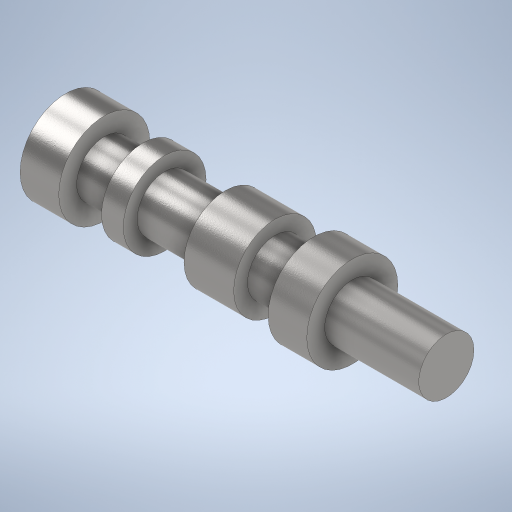
# Autodesk Inventor part: lehrerfreund
Saved by Autodesk Inventor 2024 (Build 280153000, 153)
## iProperties
Created: 2024-02-07
Part Number: lehrerfreund
Material: Stahl, galvanisiert
Document SubType Name: Modeling
Designer: ffogue
Density: 7.85 g/cm^3
Appearance: Galvanisiert
Author: ffogue
Autodesk Inventor part; units mm, degrees
ref_plane "YZ Plane" through (0, 0, 0) normal (1, 0, 0) x (0, 1, 0)
ref_plane "XZ Plane" through (0, 0, 0) normal (0, 1, 0) x (-1, 0, 0)
ref_plane "XY Plane" through (0, 0, 0) normal (0, 0, 1) x (1, 0, 0)
sketch "Skizze1" plane through (0, 0, 0) normal (0, 0, 1) x (1, 0, 0)
  line L0 (0, 0) -> (138, 0)
  line L1 (0, 0) -> (0, 16.5)
  line L2 (0, 16.5) -> (14, 16.5)
  line L3 (14, 16.5) -> (14, 10)
  line L4 (14, 10) -> (28, 10)
  line L5 (28, 10) -> (28, 15)
  line L6 (28, 15) -> (35.9017, 15)
  line L7 (35.9017, 15) -> (35.9017, 10)
  line L8 (35.9017, 10) -> (57.9017, 10)
  line L9 (57.9017, 10) -> (57.9017, 15)
  line L10 (57.9017, 15) -> (75.9017, 15)
  line L11 (75.9017, 15) -> (75.9017, 10)
  line L12 (75.9017, 10) -> (89.9017, 10)
  line L13 (89.9017, 10) -> (89.9017, 16.5)
  line L14 (89.9017, 16.5) -> (103.9017, 16.5)
  line L15 (103.9017, 16.5) -> (103.9017, 10)
  line L16 (103.9017, 10) -> (138, 10)
  line L17 (138, 10) -> (138, 0)
  point P0 (28, 12.5)
  point P1 (103.9017, 13.25)
  point P2 (89.9017, 13.25)
  dimension "d0" = 138
  dimension "d1" = 14
  dimension "d2" = 14
  dimension "d3" = 7.9017
  dimension "d4" = 22
  dimension "d5" = 14
  dimension "d6" = 14
  dimension "d7" = 18
  dimension "d8" = 33
  dimension "d9" = 20
  dimension "d10" = 30
  constraints: 36 end point, 11 perpendicular, 10 point on line, 3 midpoint, 1 coincident, 1 horizontal, 1 vertical
  measures "d0" distance between parallel lines of L17 L1
  measures "d1" distance between parallel lines of L3 L1
  measures "d2" distance from line of point (28, 12.5) L3
  measures "d3" distance between parallel lines of L7 L5
  measures "d4" distance between parallel lines of L9 L7
  measures "d5" distance from line of point (103.902, 13.25) L13
  measures "d6" distance from line of point (89.902, 13.25) L11
  measures "d7" distance between parallel lines of L11 L9
  measures "d8" diameter of L2 L0
  measures "d9" diameter of L4 L0
  measures "d10" diameter of L10 L0
revolve "Umdrehung1" add sketch "Skizze1" angle 360 about axis through (0, 0, 0) along (1, 0, 0)
